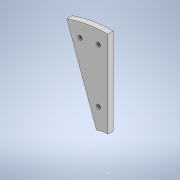
# Autodesk Inventor part: cover
Saved by Autodesk Inventor 2020.3 (Build 243373000, 373)
## iProperties
Created: 2020-11-01
Part Number: cover
Material: Generic
Document SubType Name: Modeling
Designer: Martijn
Density: 1 g/cm^3
Appearance: Default
Author: Martijn
Autodesk Inventor part; units mm, degrees
ref_plane "YZ Plane" through (0, 0, 0) normal (1, 0, 0) x (0, 1, 0)
ref_plane "XZ Plane" through (0, 0, 0) normal (0, 1, 0) x (-1, 0, 0)
ref_plane "XY Plane" through (0, 0, 0) normal (0, 0, 1) x (1, 0, 0)
sketch "Sketch1" plane through (0, 0, 0) normal (0, 0, 1) x (1, 0, 0)
  arc A0 (0, 90) -> (77.9423, -45) centre (0, 0) ccw
  arc A1 (0, 25) -> (21.6506, -12.5) centre (0, 0) ccw
  line L0 (0, 25) -> (0, 90)
  line L1 (77.9423, -45) -> (21.6506, -12.5)
  line L2 (0, 25) -> (0, 0)
  line L3 (0, 0) -> (21.6506, -12.5)
  line L4 (0, -167.6192) -> (0, 145.1192) projected
  dimension "d0" = 120
  dimension "d1" = 25
  dimension "d2" = 90
  constraints: 8 end point, 4 point on circle, 3 collinear, 2 centre point, 2 coincident
  measures "d0" angle of L1 L0
  measures "d1" radius of A1
  measures "d2" radius of A0
extrude "Extrusion1" add sketch "Sketch1" along normal blind 4 contours L0 A1 L4 A0 | L4 A1 L1 A0
sketch "Sketch2" plane through (0, 0, 0) normal (0, 0, -1) x (-1, 0, 0)
  circle A0 centre (6.9725, 79.6956) radius 1.5
  circle A1 centre (20.7055, 77.2741) radius 1.5
  circle A2 centre (6.9459, 39.3923) radius 1.5
  line L0 (6.9725, 79.6956) -> (0, 0)
  line L1 (0, 0) -> (6.9459, 39.3923)
  line L2 (20.7055, 77.2741) -> (0, 0)
  line L3 (0, 25) -> (0, 90) projected
  dimension "d14" = 3
  dimension "d15" = 3
  dimension "d16" = 3
  dimension "d17" = 80
  dimension "d18" = 80
  dimension "d19" = 40
  dimension "d20" = 10
  dimension "d21" = 5
  dimension "d22" = 15
  constraints: 6 end point, 3 centre point
  measures "d14" diameter of A1
  measures "d15" diameter of A2
  measures "d16" diameter of A0
  measures "d17" distance of L0.start L0.end
  measures "d18" distance of L2.start L0.end
  measures "d19" distance of L0.end L1.end
  measures "d20" angle of L3 L1
  measures "d21" angle of L3 L0
  measures "d22" angle of L3 L2
extrude "Extrusion2" cut sketch "Sketch2" against normal blind 10
pattern_circular "Circular Pattern1" count 12 over 220 about axis through (0, 0, 0) along (0, 0, 1) of "Extrusion2"
sketch "Sketch3" plane through (0, 0, 4) normal (0, 0, 1) x (1, 0, 0)
  point P0 (0, 0)
sketch "Sketch4" plane through (0, 0, 4) normal (0, 0, 1) x (1, 0, 0)
  arc A0 (0, 25) -> (21.6506, -12.5) centre (0, 0) ccw projected
  line L0 (0, 0) -> (-30.7818, 84.5723)
  line L1 (0, 25) -> (0, 90) projected
  line L2 (0, 0) -> (77.9423, -45)
  arc A1 (-30.7818, 84.5723) -> (77.9423, -45) centre (0, 0) ccw
  point P0 (21.6506, -12.5)
  point P1 (-8.5505, 23.4923)
  dimension "d29" = 20
  constraints: 4 end point, 3 coincident, 2 point on circle, 1 centre point
  measures "d29" angle of L1 L0
extrude "Extrusion3" cut sketch "Sketch4" against normal blind 10 contours A0 L2 A1 L0
body "Solid1"
